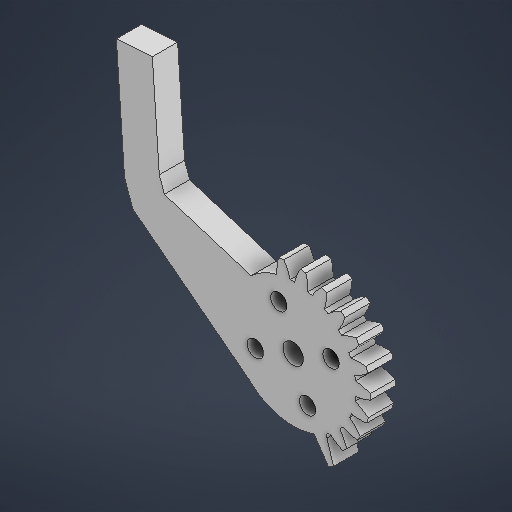
# Autodesk Inventor part: писюн 2
Saved by Autodesk Inventor 2025 (Build 290162000, 162)
## iProperties
Created: 2024-12-28
Part Number: писюн 2
Material: Типовые
Document SubType Name: Modeling
Designer: Phantom
Density: 1 g/cm^3
Appearance: По умолчанию
Author: Phantom
Autodesk Inventor part; units mm, degrees
(part 1 of 4)
ref_plane "YZ Plane" through (0, 0, 0) normal (1, 0, 0) x (0, 1, 0)
ref_plane "XZ Plane" through (0, 0, 0) normal (0, 1, 0) x (-1, 0, 0)
ref_plane "XY Plane" through (0, 0, 0) normal (0, 0, 1) x (1, 0, 0)
sketch "Эскиз1" plane through (0, 0, 0) normal (0, 0, 1) x (1, 0, 0)
  arc A0 (25.3405, 9.161) -> (8.4316, -5.5092) centre (48.8211, -34.9827) ccw
  arc A1 (16.1963, 14.3431) -> (25.3405, 9.161) centre (40.8164, 47.1281) ccw
  arc A2 (16.1963, 14.3431) -> (-11.1891, 14.3431) centre (2.5036, -3.8906) ccw
  line L0 (-11.1891, 14.3431) -> (-11.0924, 14.1698)
  line L1 (-11.0924, 14.1698) -> (-10.8798, 13.8428)
  line L2 (-10.8798, 13.8428) -> (-10.6476, 13.5415)
  line L3 (-10.6476, 13.5415) -> (-10.3902, 13.2744)
  line L4 (-10.3902, 13.2744) -> (-10.0964, 13.0589)
  line L5 (-10.0964, 13.0589) -> (-9.8198, 12.8188)
  line L6 (-9.8198, 12.8188) -> (-9.6918, 12.6838)
  line L7 (-9.6918, 12.6838) -> (-9.5723, 12.5363)
  line L8 (-9.5723, 12.5363) -> (-9.4633, 12.3731)
  line L9 (-9.4633, 12.3731) -> (-9.3681, 12.1883)
  line L10 (-9.3681, 12.1883) -> (-9.3278, 12.0845)
  line L11 (-9.3278, 12.0845) -> (-9.2943, 11.9695)
  line L12 (-9.2943, 11.9695) -> (-9.2712, 11.8376)
  line L13 (-9.2712, 11.8376) -> (-9.2668, 11.6743)
  line L14 (-9.2668, 11.6743) -> (-9.3696, 11.329)
  line L15 (-9.3696, 11.329) -> (-9.7265, 10.6764)
  line L16 (-9.7265, 10.6764) -> (-10.0432, 10.0032)
  line L17 (-10.0432, 10.0032) -> (-10.2615, 9.7167)
  line L18 (-10.2615, 9.7167) -> (-10.3959, 9.6239)
  line L19 (-10.3959, 9.6239) -> (-10.5161, 9.5649)
  line L20 (-10.5161, 9.5649) -> (-10.6287, 9.5241)
  line L21 (-10.6287, 9.5241) -> (-10.7364, 9.4955)
  line L22 (-10.7364, 9.4955) -> (-10.9417, 9.4634)
  line L23 (-10.9417, 9.4634) -> (-11.1379, 9.4552)
  line L24 (-11.1379, 9.4552) -> (-11.3274, 9.4648)
  line L25 (-11.3274, 9.4648) -> (-11.5119, 9.4885)
  line L26 (-11.5119, 9.4885) -> (-11.8689, 9.5704)
  line L27 (-11.8689, 9.5704) -> (-12.2162, 9.6807)
  line L28 (-12.2162, 9.6807) -> (-12.5837, 9.731)
  line L29 (-12.5837, 9.731) -> (-12.964, 9.741)
  line L30 (-12.964, 9.741) -> (-13.3534, 9.7199)
  line L31 (-13.3534, 9.7199) -> (-13.7498, 9.6714)
  line L32 (-13.7498, 9.6714) -> (-14.1519, 9.5976)
  line L33 (-14.1519, 9.5976) -> (-14.5586, 9.4998)
  line L34 (-14.5586, 9.4998) -> (-14.9687, 9.3787)
  line L35 (-14.9687, 9.3787) -> (-15.3815, 9.2349)
  line L36 (-15.3815, 9.2349) -> (-15.796, 9.069)
  line L37 (-15.796, 9.069) -> (-16.1075, 8.9301)
  line L38 (-16.1075, 8.9301) -> (-16.4414, 6.8067)
  line L39 (-16.4414, 6.8067) -> (-16.1875, 6.579)
  line L40 (-16.1875, 6.579) -> (-15.8439, 6.2938)
  line L41 (-15.8439, 6.2938) -> (-15.4952, 6.0303)
  line L42 (-15.4952, 6.0303) -> (-15.142, 5.7892)
  line L43 (-15.142, 5.7892) -> (-14.785, 5.5713)
  line L44 (-14.785, 5.5713) -> (-14.425, 5.3776)
  line L45 (-14.425, 5.3776) -> (-14.0625, 5.2099)
  line L46 (-14.0625, 5.2099) -> (-13.6984, 5.0703)
  line L47 (-13.6984, 5.0703) -> (-13.3334, 4.963)
  line L48 (-13.3334, 4.963) -> (-12.9682, 4.8982)
  line L49 (-12.9682, 4.8982) -> (-12.6038, 4.8965)
  line L50 (-12.6038, 4.8965) -> (-12.2389, 4.8649)
  line L51 (-12.2389, 4.8649) -> (-12.056, 4.8309)
  line L52 (-12.056, 4.8309) -> (-11.8727, 4.7818)
  line L53 (-11.8727, 4.7818) -> (-11.6885, 4.7139)
  line L54 (-11.6885, 4.7139) -> (-11.5029, 4.6203)
  line L55 (-11.5029, 4.6203) -> (-11.4093, 4.56)
  line L56 (-11.4093, 4.56) -> (-11.3146, 4.4866)
  line L57 (-11.3146, 4.4866) -> (-11.2183, 4.3936)
  line L58 (-11.2183, 4.3936) -> (-11.1188, 4.264)
  line L59 (-11.1188, 4.264) -> (-10.999, 3.9243)
  line L60 (-10.999, 3.9243) -> (-10.9042, 3.1865)
  line L61 (-10.9042, 3.1865) -> (-10.7647, 2.4558)
  line L62 (-10.7647, 2.4558) -> (-10.7729, 2.0956)
  line L63 (-10.7729, 2.0956) -> (-10.8272, 1.9416)
  line L64 (-10.8272, 1.9416) -> (-10.8897, 1.8232)
  line L65 (-10.8897, 1.8232) -> (-10.9568, 1.724)
  line L66 (-10.9568, 1.724) -> (-11.0271, 1.6375)
  line L67 (-11.0271, 1.6375) -> (-11.1743, 1.4909)
  line L68 (-11.1743, 1.4909) -> (-11.3282, 1.369)
  line L69 (-11.3282, 1.369) -> (-11.4872, 1.2653)
  line L70 (-11.4872, 1.2653) -> (-11.6504, 1.1761)
  line L71 (-11.6504, 1.1761) -> (-11.9874, 1.0325)
  line L72 (-11.9874, 1.0325) -> (-12.3332, 0.9175)
  line L73 (-12.3332, 0.9175) -> (-12.66, 0.7423)
  line L74 (-12.66, 0.7423) -> (-12.9736, 0.5268)
  line L75 (-12.9736, 0.5268) -> (-13.2762, 0.2808)
  line L76 (-13.2762, 0.2808) -> (-13.5684, 0.0086)
  line L77 (-13.5684, 0.0086) -> (-13.8504, -0.2874)
  line L78 (-13.8504, -0.2874) -> (-14.1218, -0.6056)
  line L79 (-14.1218, -0.6056) -> (-14.3824, -0.9447)
  line L80 (-14.3824, -0.9447) -> (-14.6319, -1.3036)
  line L81 (-14.6319, -1.3036) -> (-14.8697, -1.6815)
  line L82 (-14.8697, -1.6815) -> (-15.0401, -1.9769)
  line L83 (-15.0401, -1.9769) -> (-14.0621, -3.891)
  line L84 (-14.0621, -3.891) -> (-13.7228, -3.9261)
  line L85 (-13.7228, -3.9261) -> (-13.2773, -3.9548)
  line L86 (-13.2773, -3.9548) -> (-12.8403, -3.963)
  line L87 (-12.8403, -3.963) -> (-12.4128, -3.9505)
  line L88 (-12.4128, -3.9505) -> (-11.9959, -3.917)
  line L89 (-11.9959, -3.917) -> (-11.5908, -3.862)
  line L90 (-11.5908, -3.862) -> (-11.199, -3.7847)
  line L91 (-11.199, -3.7847) -> (-10.8224, -3.6836)
  line L92 (-10.8224, -3.6836) -> (-10.464, -3.5558)
  line L93 (-10.464, -3.5558) -> (-10.1304, -3.3936)
  line L94 (-10.1304, -3.3936) -> (-9.8347, -3.1808)
  line L95 (-9.8347, -3.1808) -> (-9.5209, -2.9918)
  line L96 (-9.5209, -2.9918) -> (-9.353, -2.9118)
  line L97 (-9.353, -2.9118) -> (-9.1758, -2.8438)
  line L98 (-9.1758, -2.8438) -> (-8.9868, -2.7905)
  line L99 (-8.9868, -2.7905) -> (-8.7817, -2.7571)
  line L100 (-8.7817, -2.7571) -> (-8.6705, -2.7509)
  line L101 (-8.6705, -2.7509) -> (-8.5508, -2.7546)
  line L102 (-8.5508, -2.7546) -> (-8.4182, -2.7733)
  line L103 (-8.4182, -2.7733) -> (-8.2615, -2.8196)
  line L104 (-8.2615, -2.8196) -> (-7.9649, -3.024)
  line L105 (-7.9649, -3.024) -> (-7.4545, -3.5652)
  line L106 (-7.4545, -3.5652) -> (-6.9122, -4.0744)
  line L107 (-6.9122, -4.0744) -> (-6.7071, -4.3705)
  line L108 (-6.7071, -4.3705) -> (-6.6604, -4.5271)
  line L109 (-6.6604, -4.5271) -> (-6.6415, -4.6596)
  line L110 (-6.6415, -4.6596) -> (-6.6374, -4.7793)
  line L111 (-6.6374, -4.7793) -> (-6.6435, -4.8906)
  line L112 (-6.6435, -4.8906) -> (-6.6764, -5.0958)
  line L113 (-6.6764, -5.0958) -> (-6.7292, -5.2848)
  line L114 (-6.7292, -5.2848) -> (-6.7969, -5.4622)
  line L115 (-6.7969, -5.4622) -> (-6.8765, -5.6303)
  line L116 (-6.8765, -5.6303) -> (-7.0647, -5.9445)
  line L117 (-7.0647, -5.9445) -> (-7.2769, -6.2407)
  line L118 (-7.2769, -6.2407) -> (-7.4384, -6.5746)
  line L119 (-7.4384, -6.5746) -> (-7.5654, -6.9333)
  line L120 (-7.5654, -6.9333) -> (-7.6656, -7.3102)
  line L121 (-7.6656, -7.3102) -> (-7.742, -7.7022)
  line L122 (-7.742, -7.7022) -> (-7.7961, -8.1074)
  line L123 (-7.7961, -8.1074) -> (-7.8287, -8.5243)
  line L124 (-7.8287, -8.5243) -> (-7.8403, -8.9518)
  line L125 (-7.8403, -8.9518) -> (-7.8311, -9.3888)
  line L126 (-7.8311, -9.3888) -> (-7.8013, -9.8343)
  line L127 (-7.8013, -9.8343) -> (-7.7656, -10.1735)
  line L128 (-7.7656, -10.1735) -> (-5.8492, -11.1472)
  line L129 (-5.8492, -11.1472) -> (-5.5542, -10.9761)
  line L130 (-5.5542, -10.9761) -> (-5.1768, -10.7375)
  line L131 (-5.1768, -10.7375) -> (-4.8185, -10.4872)
  line L132 (-4.8185, -10.4872) -> (-4.48, -10.2258)
  line L133 (-4.48, -10.2258) -> (-4.1624, -9.9537)
  line L134 (-4.1624, -9.9537) -> (-3.867, -9.6711)
  line L135 (-3.867, -9.6711) -> (-3.5955, -9.3782)
  line L136 (-3.5955, -9.3782) -> (-3.3502, -9.0751)
  line L137 (-3.3502, -9.0751) -> (-3.1354, -8.7611)
  line L138 (-3.1354, -8.7611) -> (-2.9609, -8.4338)
  line L139 (-2.9609, -8.4338) -> (-2.8467, -8.0877)
  line L140 (-2.8467, -8.0877) -> (-2.7039, -7.7505)
  line L141 (-2.7039, -7.7505) -> (-2.615, -7.5871)
  line L142 (-2.615, -7.5871) -> (-2.5117, -7.4278)
  line L143 (-2.5117, -7.4278) -> (-2.3901, -7.2737)
  line L144 (-2.3901, -7.2737) -> (-2.2438, -7.1261)
  line L145 (-2.2438, -7.1261) -> (-2.1575, -7.0556)
  line L146 (-2.1575, -7.0556) -> (-2.0585, -6.9883)
  line L147 (-2.0585, -6.9883) -> (-1.9402, -6.9255)
  line L148 (-1.9402, -6.9255) -> (-1.7863, -6.8709)
  line L149 (-1.7863, -6.8709) -> (-1.4262, -6.8619)
  line L150 (-1.4262, -6.8619) -> (-0.6951, -6.9997)
  line L151 (-0.6951, -6.9997) -> (0.0429, -7.0929)
  line L152 (0.0429, -7.0929) -> (0.3829, -7.2119)
  line L153 (0.3829, -7.2119) -> (0.5127, -7.3112)
  line L154 (0.5127, -7.3112) -> (0.6059, -7.4072)
  line L155 (0.6059, -7.4072) -> (0.6795, -7.5017)
  line L156 (0.6795, -7.5017) -> (0.74, -7.5953)
  line L157 (0.74, -7.5953) -> (0.834, -7.7806)
  line L158 (0.834, -7.7806) -> (0.9024, -7.9646)
  line L159 (0.9024, -7.9646) -> (0.9519, -8.1479)
  line L160 (0.9519, -8.1479) -> (0.9863, -8.3307)
  line L161 (0.9863, -8.3307) -> (1.0187, -8.6955)
  line L162 (1.0187, -8.6955) -> (1.0212, -9.0599)
  line L163 (1.0212, -9.0599) -> (1.0869, -9.4249)
  line L164 (1.0869, -9.4249) -> (1.1949, -9.7897)
  line L165 (1.1949, -9.7897) -> (1.3353, -10.1535)
  line L166 (1.3353, -10.1535) -> (1.5039, -10.5156)
  line L167 (1.5039, -10.5156) -> (1.6983, -10.8752)
  line L168 (1.6983, -10.8752) -> (1.9171, -11.2317)
  line L169 (1.9171, -11.2317) -> (2.159, -11.5843)
  line L170 (2.159, -11.5843) -> (2.4233, -11.9325)
  line L171 (2.4233, -11.9325) -> (2.7092, -12.2754)
  line L172 (2.7092, -12.2754) -> (2.9375, -12.5288)
  line L173 (2.9375, -12.5288) -> (5.0602, -12.1901)
  line L174 (5.0602, -12.1901) -> (5.1983, -11.8783)
  line L175 (5.1983, -11.8783) -> (5.3633, -11.4634)
  line L176 (5.3633, -11.4634) -> (5.5062, -11.0504)
  line L177 (5.5062, -11.0504) -> (5.6263, -10.6399)
  line L178 (5.6263, -10.6399) -> (5.7233, -10.2331)
  line L179 (5.7233, -10.2331) -> (5.7962, -9.8308)
  line L180 (5.7962, -9.8308) -> (5.8437, -9.4343)
  line L181 (5.8437, -9.4343) -> (5.864, -9.0449)
  line L182 (5.864, -9.0449) -> (5.8532, -8.6645)
  line L183 (5.8532, -8.6645) -> (5.802, -8.2972)
  line L184 (5.802, -8.2972) -> (5.691, -7.9502)
  line L185 (5.691, -7.9502) -> (5.6083, -7.5933)
  line L186 (5.6083, -7.5933) -> (5.5841, -7.4089)
  line L187 (5.5841, -7.4089) -> (5.5741, -7.2193)
  line L188 (5.5741, -7.2193) -> (5.5818, -7.0232)
  line L189 (5.5818, -7.0232) -> (5.6135, -6.8178)
  line L190 (5.6135, -6.8178) -> (5.6419, -6.7101)
  line L191 (5.6419, -6.7101) -> (5.6824, -6.5974)
  line L192 (5.6824, -6.5974) -> (5.7412, -6.4771)
  line L193 (5.7412, -6.4771) -> (5.8336, -6.3424)
  line L194 (5.8336, -6.3424) -> (6.1197, -6.1235)
  line L195 (6.1197, -6.1235) -> (6.7921, -5.8052)
  line L196 (6.7921, -5.8052) -> (7.444, -5.4468)
  line L197 (7.444, -5.4468) -> (7.789, -5.3433)
  line L198 (7.789, -5.3433) -> (7.9523, -5.3473)
  line L199 (7.9523, -5.3473) -> (8.0842, -5.3702)
  line L200 (8.0842, -5.3702) -> (8.1993, -5.4034)
  line L201 (8.1993, -5.4034) -> (8.3032, -5.4435)
  line L202 (8.3032, -5.4435) -> (8.4316, -5.5092)
  circle A3 centre (-5.9559, 8.675) radius 1.6
  circle A4 centre (-2.3455, -2.0471) radius 1.6
  circle A5 centre (8.3767, 1.5633) radius 1.6
  circle A6 centre (4.7663, 12.2855) radius 1.6
  circle A7 centre (1.2104, 5.1192) radius 2.5
  line L203 (-13.3615, -49.398) -> (-13.2922, -49.3107)
  line L204 (-13.2922, -49.3107) -> (-13.2099, -49.2238)
  line L205 (-13.2099, -49.2238) -> (-13.1078, -49.1372)
  line L206 (-9.6165, -50.932) -> (-9.433, -51.2653)
  line L207 (-9.433, -51.2653) -> (-9.3025, -51.4628)
  line L208 (-9.7587, -50.5894) -> (-9.6165, -50.932)
  line L209 (-10.4254, -49.1402) -> (-10.3463, -49.2187)
  line L210 (-10.3463, -49.2187) -> (-10.2149, -49.3797)
  line L211 (-10.2149, -49.3797) -> (-10.1088, -49.5448)
  line L212 (-10.1088, -49.5448) -> (-10.0213, -49.7133)
  line L213 (-10.0213, -49.7133) -> (-9.9486, -49.8845)
  line L214 (-9.9486, -49.8845) -> (-9.8389, -50.234)
  line L215 (-9.8389, -50.234) -> (-9.7587, -50.5894)
  circle A8 centre (-5.8233, -40.9429) radius 1.6
  arc A9 (11.8073, -35.0555) -> (-9.3025, -51.4628) centre (30.819, -81.3) ccw
  line L216 (-13.8831, -51.1857) -> (-13.7825, -50.8287)
  line L217 (-13.7825, -50.8287) -> (-13.7449, -50.4663)
  line L218 (-13.7449, -50.4663) -> (-13.6775, -50.1063)
  line L219 (-13.6775, -50.1063) -> (-13.6256, -49.9276)
  line L220 (-13.6256, -49.9276) -> (-13.5587, -49.75)
  line L221 (-13.5587, -49.75) -> (-13.4729, -49.5734)
  line L222 (-13.4729, -49.5734) -> (-13.3615, -49.398)
  line L223 (-11.1347, -48.8769) -> (-10.7771, -48.9205)
  line L224 (-11.8756, -48.9436) -> (-11.1347, -48.8769)
  line L225 (-12.6192, -48.9652) -> (-11.8756, -48.9436)
  line L226 (-10.7771, -48.9205) -> (-10.6291, -48.9898)
  line L227 (-10.6291, -48.9898) -> (-10.5175, -49.0637)
  line L228 (-10.5175, -49.0637) -> (-10.4254, -49.1402)
  line L229 (-13.1078, -49.1372) -> (-12.9691, -49.0509)
  line L230 (-12.9691, -49.0509) -> (-12.6192, -48.9652)
  line L231 (-15.7727, -53.8665) -> (-15.455, -53.5527)
  line L232 (-15.455, -53.5527) -> (-15.1584, -53.2317)
  line L233 (-15.1584, -53.2317) -> (-14.8836, -52.904)
  line L234 (-14.8836, -52.904) -> (-14.6315, -52.5703)
  line L235 (-14.0258, -51.5384) -> (-13.8831, -51.1857)
  line L236 (-14.2006, -51.887) -> (-14.0258, -51.5384)
  line L237 (-14.4034, -52.2311) -> (-14.2006, -51.887)
  line L238 (-14.6315, -52.5703) -> (-14.4034, -52.2311)
  line L239 (-16.0243, -54.0967) -> (-15.7727, -53.8665)
  line L240 (-18.165, -48.7455) -> (-18.2068, -48.9267)
  line L241 (-18.2068, -48.9267) -> (-18.3236, -49.2739)
  line L242 (-18.3236, -49.2739) -> (-18.4675, -49.6086)
  line L243 (-18.4675, -49.6086) -> (-18.5539, -49.9694)
  line L244 (-18.5539, -49.9694) -> (-18.6013, -50.3469)
  line L245 (-18.1045, -53.555) -> (-16.0243, -54.0967)
  line L246 (-18.2119, -53.2313) -> (-18.1045, -53.555)
  line L247 (-18.3362, -52.8024) -> (-18.2119, -53.2313)
  line L248 (-18.4385, -52.3775) -> (-18.3362, -52.8024)
  line L249 (-18.5186, -51.9574) -> (-18.4385, -52.3775)
  line L250 (-18.5758, -51.5431) -> (-18.5186, -51.9574)
  line L251 (-18.6096, -51.1357) -> (-18.5758, -51.5431)
  line L252 (-18.6013, -50.3469) -> (-18.6187, -50.7364)
  line L253 (-18.6187, -50.7364) -> (-18.6096, -51.1357)
  line L254 (-19.827, -46.6133) -> (-19.2128, -47.0328)
  line L255 (-19.2128, -47.0328) -> (-18.5742, -47.4144)
  line L256 (-18.5742, -47.4144) -> (-18.3105, -47.6599)
  line L257 (-18.3105, -47.6599) -> (-18.2315, -47.8028)
  line L258 (-18.2315, -47.8028) -> (-18.1846, -47.9283)
  line L259 (-18.1846, -47.9283) -> (-18.1551, -48.0444)
  line L260 (-18.1551, -48.0444) -> (-18.1373, -48.1543)
  line L261 (-18.1373, -48.1543) -> (-18.1256, -48.3618)
  line L262 (-18.1256, -48.3618) -> (-18.1368, -48.5578)
  line L263 (-18.1368, -48.5578) -> (-18.165, -48.7455)
  line L264 (-24.325, -43.2978) -> (-24.6235, -43.5101)
  line L265 (-24.1846, -43.1758) -> (-24.325, -43.2978)
  line L266 (-24.0514, -43.0405) -> (-24.1846, -43.1758)
  line L267 (-23.9271, -42.8885) -> (-24.0514, -43.0405)
  line L268 (-23.8146, -42.7138) -> (-23.9271, -42.8885)
  line L269 (-23.7645, -42.6143) -> (-23.8146, -42.7138)
  line L270 (-23.7201, -42.5031) -> (-23.7645, -42.6143)
  line L271 (-23.6843, -42.3741) -> (-23.7201, -42.5031)
  line L272 (-23.6642, -42.2119) -> (-23.6843, -42.3741)
  line L273 (-26.3323, -35.144) -> (-26.6951, -35.1105)
  line L274 (-25.966, -35.1478) -> (-26.3323, -35.144)
  line L275 (-25.7807, -35.1315) -> (-25.966, -35.1478)
  line L276 (-25.5935, -35.1004) -> (-25.7807, -35.1315)
  line L277 (-25.4036, -35.0505) -> (-25.5935, -35.1004)
  line L278 (-25.2099, -34.9752) -> (-25.4036, -35.0505)
  line L279 (-25.1108, -34.9243) -> (-25.2099, -34.9752)
  line L280 (-25.0095, -34.8603) -> (-25.1108, -34.9243)
  line L281 (-22.4775, -47.8682) -> (-22.1548, -47.6668)
  line L282 (-22.1548, -47.6668) -> (-21.8636, -47.4371)
  line L283 (-25.6882, -39.8199) -> (-25.5023, -39.814)
  line L284 (-26.0514, -39.867) -> (-25.6882, -39.8199)
  line L285 (-26.7783, -39.958) -> (-26.4077, -39.9433)
  line L286 (-26.4077, -39.9433) -> (-26.0514, -39.867)
  line L287 (-25.5023, -39.814) -> (-25.3126, -39.8228)
  line L288 (-25.3126, -39.8228) -> (-25.1182, -39.8498)
  line L289 (-25.1182, -39.8498) -> (-24.9169, -39.9016)
  line L290 (-24.9169, -39.9016) -> (-24.8125, -39.9405)
  line L291 (-24.8125, -39.9405) -> (-24.7044, -39.9919)
  line L292 (-24.7044, -39.9919) -> (-24.5904, -40.0623)
  line L293 (-24.5904, -40.0623) -> (-24.4655, -40.1675)
  line L294 (-24.4655, -40.1675) -> (-24.2759, -40.4738)
  line L295 (-24.2759, -40.4738) -> (-24.0256, -41.1743)
  line L296 (-24.0256, -41.1743) -> (-23.7332, -41.8584)
  line L297 (-23.7332, -41.8584) -> (-23.6642, -42.2119)
  line L298 (-24.2664, -32.892) -> (-24.4757, -33.6058)
  line L299 (-24.2398, -32.5327) -> (-24.2664, -32.892)
  line L300 (-24.279, -32.3741) -> (-24.2398, -32.5327)
  line L301 (-24.3298, -32.2502) -> (-24.279, -32.3741)
  line L302 (-24.3871, -32.145) -> (-24.3298, -32.2502)
  line L303 (-24.4487, -32.0522) -> (-24.3871, -32.145)
  line L304 (-24.5811, -31.892) -> (-24.4487, -32.0522)
  line L305 (-24.8708, -31.6373) -> (-24.7225, -31.7559)
  line L306 (-24.7225, -31.7559) -> (-24.5811, -31.892)
  circle A10 centre (-19.3845, -32.452) radius 1.6
  arc A11 (3.2188, -28.9967) -> (-27.6302, -28.9967) centre (-12.2057, -45.7908) ccw
  circle A12 centre (-8.3584, -29.9169) radius 1.6
  line L307 (-24.9367, -43.6962) -> (-25.2186, -43.9373)
  line L308 (-25.2186, -43.9373) -> (-25.4788, -44.2149)
  line L309 (-25.4788, -44.2149) -> (-25.7219, -44.5198)
  line L310 (-25.7219, -44.5198) -> (-25.9492, -44.8482)
  line L311 (-25.9492, -44.8482) -> (-26.1614, -45.1976)
  line L312 (-26.1614, -45.1976) -> (-26.3585, -45.5664)
  line L313 (-26.3585, -45.5664) -> (-26.5407, -45.9534)
  line L314 (-24.6235, -43.5101) -> (-24.9367, -43.6962)
  line L315 (-27.0648, -35.1399) -> (-27.4385, -35.2114)
  line L316 (-24.9047, -34.777) -> (-25.0095, -34.8603)
  line L317 (-24.7932, -34.6577) -> (-24.9047, -34.777)
  line L318 (-24.6412, -34.3311) -> (-24.7932, -34.6577)
  line L319 (-28.3264, -39.674) -> (-27.9333, -39.7862)
  circle A13 centre (-12.6039, -36.6975) radius 2.5
  line L320 (-26.6951, -35.1105) -> (-27.0648, -35.1399)
  line L321 (-22.8239, -48.0475) -> (-22.4775, -47.8682)
  line L322 (-23.1901, -48.2067) -> (-22.8239, -48.0475)
  line L323 (-23.5741, -48.347) -> (-23.1901, -48.2067)
  line L324 (-23.9742, -48.4688) -> (-23.5741, -48.347)
  line L325 (-24.3891, -48.5724) -> (-23.9742, -48.4688)
  line L326 (-24.8178, -48.6578) -> (-24.3891, -48.5724)
  line L327 (-25.2592, -48.7249) -> (-24.8178, -48.6578)
  line L328 (-26.7077, -46.3573) -> (-26.8592, -46.7773)
  line L329 (-26.8592, -46.7773) -> (-26.9625, -47.1023)
  line L330 (-26.9625, -47.1023) -> (-25.5981, -48.7632)
  line L331 (-25.5981, -48.7632) -> (-25.2592, -48.7249)
  line L332 (-24.4757, -33.6058) -> (-24.6412, -34.3311)
  line L333 (-27.4385, -35.2114) -> (-27.8144, -35.3153)
  line L334 (-27.8144, -35.3153) -> (-28.1913, -35.4473)
  line L335 (-28.5684, -35.6053) -> (-28.9447, -35.7878)
  line L336 (-28.9447, -35.7878) -> (-29.3195, -35.9938)
  line L337 (-29.3195, -35.9938) -> (-29.692, -36.2224)
  line L338 (-29.692, -36.2224) -> (-30.0614, -36.4731)
  line L339 (-30.0614, -36.4731) -> (-30.3361, -36.6753)
  line L340 (-28.1913, -35.4473) -> (-28.5684, -35.6053)
  line L341 (-25.0246, -31.5328) -> (-24.8708, -31.6373)
  line L342 (-25.3462, -31.3574) -> (-25.0246, -31.5328)
  line L343 (-25.9877, -31.0037) -> (-25.6793, -31.2097)
  line L344 (-26.279, -30.759) -> (-25.9877, -31.0037)
  line L345 (-26.5565, -30.485) -> (-26.279, -30.759)
  line L346 (-26.8212, -30.1859) -> (-26.5565, -30.485)
  line L347 (-27.0732, -29.864) -> (-26.8212, -30.1859)
  line L348 (-27.3127, -29.5212) -> (-27.0732, -29.864)
  line L349 (-27.5395, -29.1586) -> (-27.3127, -29.5212)
  line L350 (-27.6302, -28.9967) -> (-27.5395, -29.1586)
  line L351 (-25.6793, -31.2097) -> (-25.3462, -31.3574)
  line L352 (-30.3361, -36.6753) -> (-30.2085, -38.8211)
  line L353 (-30.2085, -38.8211) -> (-29.9118, -38.9893)
  line L354 (-29.9118, -38.9893) -> (-29.5152, -39.1944)
  line L355 (-29.5152, -39.1944) -> (-29.1183, -39.3773)
  line L356 (-29.1183, -39.3773) -> (-28.7217, -39.5374)
  line L357 (-28.7217, -39.5374) -> (-28.3264, -39.674)
  line L358 (-27.9333, -39.7862) -> (-27.5434, -39.8726)
  line L359 (-27.5434, -39.8726) -> (-27.1579, -39.9312)
  line L360 (-26.5407, -45.9534) -> (-26.7077, -46.3573)
  line L361 (-27.1579, -39.9312) -> (-26.7783, -39.958)
  line L362 (-21.8636, -47.4371) -> (-21.6201, -47.166)
  line L363 (-21.6201, -47.166) -> (-21.354, -46.9143)
  line L364 (-21.354, -46.9143) -> (-21.207, -46.8003)
  line L365 (-21.207, -46.8003) -> (-21.0484, -46.696)
  line L366 (-21.0484, -46.696) -> (-20.8752, -46.6035)
  line L367 (-20.682, -46.5271) -> (-20.5747, -46.4972)
  circle A14 centre (-16.8493, -43.478) radius 1.6
  line L368 (-20.1605, -46.4769) -> (-19.827, -46.6133)
  line L369 (-20.3234, -46.4652) -> (-20.1605, -46.4769)
  line L370 (-20.4569, -46.4753) -> (-20.3234, -46.4652)
  line L371 (-20.5747, -46.4972) -> (-20.4569, -46.4753)
  line L372 (-20.8752, -46.6035) -> (-20.682, -46.5271)
  arc A15 (3.2188, -28.9967) -> (11.8073, -35.0555) centre (30.9527, 1.1999) ccw
  point P0 (0, 0)
  point P1 (-20.9679, -17.3277)
  point P2 (-6.0215, -34.9827)
  constraints: 746 end point, 16 centre point, 12 point on circle
extrude "Выдавливание1" add sketch "Эскиз1" along normal blind 5 contours L222 L221 L220 L219 L218 L217 L216 L235 L236 L237 L238 L234 L233 L232 L231 L239 L245 L246 L247 L248 L249 L250 L251 L253 L252 L244 L243 L242 L241 L240 L263 L262 L261 L260 L259 L258 L257 L256 L255 L254 L368 L369 L370 L371 L367 L372 L366 L365 L364 L363 L362 L282 L281 L321 L322 L323 L324 L325 L326 L327 L331 L330 L329 L328 L360 L313 L312 L311 L310 L309 L308 L307 L314 L264 L265 L266 L267 L268 L269 L270 L271 L272 L297 L296 L295 L294 L293 L292 L291 L290 L289 L288 L287 L283 L284 L286 L285 L361 L359 L358 L319 L357 L356 L355 L354 L353 L352 L339 L338 L337 L336 L335 L340 L334 L333 L315 L320 L273 L274 L275 L276 L277 L278 L279 L280 L316 L317 L318 L332 L298 L299 L300 L301 L302 L303 L304 L306 L305 L341 L342 L351 L343 L344 L345 L346 L347 L348 L349 L350 A11 A15 A9 L207 L206 L208 L215 L214 L213 L212 L211 L210 L209 L228 L227 L226 L223 L224 L225 L230 L229 L205 L204 L203
sketch "Эскиз2" plane through (0, 0, 0) normal (0, 0, -1) x (-1, 0, 0)
  line L0 (-8.3032, -5.4435) -> (-8.4316, -5.5092) projected
  line L1 (-8.4316, -5.5092) -> (-25.3405, -5.5092)
  line L2 (11.1891, 14.3431) -> (11.0924, 14.1698) projected
  arc A0 (11.1891, 14.3431) -> (-16.1963, 14.3431) centre (-2.5036, -3.8906) ccw projected
  arc A1 (-25.3405, 9.161) -> (-16.1963, 14.3431) centre (-40.8164, 47.1281) ccw projected
  arc A2 (-8.4316, -5.5092) -> (-25.3405, 9.161) centre (-48.8211, -34.9827) ccw projected
  line L3 (-8.3032, -5.4435) -> (-8.4316, -5.5092) projected
  line L4 (-8.1993, -5.4034) -> (-8.3032, -5.4435) projected
  line L5 (-8.0842, -5.3702) -> (-8.1993, -5.4034) projected
  line L6 (-7.9523, -5.3473) -> (-8.0842, -5.3702) projected
  line L7 (-7.789, -5.3433) -> (-7.9523, -5.3473) projected
  line L8 (-7.444, -5.4468) -> (-7.789, -5.3433) projected
  line L9 (-6.7921, -5.8052) -> (-7.444, -5.4468) projected
  line L10 (-6.1197, -6.1235) -> (-6.7921, -5.8052) projected
  line L11 (-5.8336, -6.3424) -> (-6.1197, -6.1235) projected
  line L12 (-5.7412, -6.4771) -> (-5.8336, -6.3424) projected
  line L13 (-5.6824, -6.5974) -> (-5.7412, -6.4771) projected
  line L14 (-5.6419, -6.7101) -> (-5.6824, -6.5974) projected
  line L15 (-5.6135, -6.8178) -> (-5.6419, -6.7101) projected
  line L16 (-5.5818, -7.0232) -> (-5.6135, -6.8178) projected
  line L17 (-5.5741, -7.2193) -> (-5.5818, -7.0232) projected
  line L18 (-5.5841, -7.4089) -> (-5.5741, -7.2193) projected
  line L19 (-5.6083, -7.5933) -> (-5.5841, -7.4089) projected
  line L20 (-5.691, -7.9502) -> (-5.6083, -7.5933) projected
  line L21 (-5.802, -8.2972) -> (-5.691, -7.9502) projected
  line L22 (-5.8532, -8.6645) -> (-5.802, -8.2972) projected
  line L23 (-5.864, -9.0449) -> (-5.8532, -8.6645) projected
  line L24 (-5.8437, -9.4343) -> (-5.864, -9.0449) projected
  line L25 (-5.7962, -9.8308) -> (-5.8437, -9.4343) projected
  line L26 (-5.7233, -10.2331) -> (-5.7962, -9.8308) projected
  line L27 (-5.6263, -10.6399) -> (-5.7233, -10.2331) projected
  line L28 (-5.5062, -11.0504) -> (-5.6263, -10.6399) projected
  line L29 (-5.3633, -11.4634) -> (-5.5062, -11.0504) projected
  line L30 (-5.1983, -11.8783) -> (-5.3633, -11.4634) projected
  line L31 (-5.0602, -12.1901) -> (-5.1983, -11.8783) projected
  line L32 (-2.9375, -12.5288) -> (-5.0602, -12.1901) projected
  line L33 (-2.7092, -12.2754) -> (-2.9375, -12.5288) projected
  line L34 (-2.4233, -11.9325) -> (-2.7092, -12.2754) projected
  line L35 (-2.159, -11.5843) -> (-2.4233, -11.9325) projected
  line L36 (-1.9171, -11.2317) -> (-2.159, -11.5843) projected
  line L37 (-1.6983, -10.8752) -> (-1.9171, -11.2317) projected
  line L38 (-1.5039, -10.5156) -> (-1.6983, -10.8752) projected
  line L39 (-1.3353, -10.1535) -> (-1.5039, -10.5156) projected
  line L40 (-1.1949, -9.7897) -> (-1.3353, -10.1535) projected
  line L41 (-1.0869, -9.4249) -> (-1.1949, -9.7897) projected
  line L42 (-1.0212, -9.0599) -> (-1.0869, -9.4249) projected
  line L43 (-1.0187, -8.6955) -> (-1.0212, -9.0599) projected
  line L44 (-0.9863, -8.3307) -> (-1.0187, -8.6955) projected
  line L45 (-0.9519, -8.1479) -> (-0.9863, -8.3307) projected
  line L46 (-0.9024, -7.9646) -> (-0.9519, -8.1479) projected
  line L47 (-0.834, -7.7806) -> (-0.9024, -7.9646) projected
  line L48 (-0.74, -7.5953) -> (-0.834, -7.7806) projected
  line L49 (-0.6795, -7.5017) -> (-0.74, -7.5953) projected
  line L50 (-0.6059, -7.4072) -> (-0.6795, -7.5017) projected
  line L51 (-0.5127, -7.3112) -> (-0.6059, -7.4072) projected
  line L52 (-0.3829, -7.2119) -> (-0.5127, -7.3112) projected
  line L53 (-0.0429, -7.0929) -> (-0.3829, -7.2119) projected
  line L54 (0.6951, -6.9997) -> (-0.0429, -7.0929) projected
  line L55 (1.4262, -6.8619) -> (0.6951, -6.9997) projected
  line L56 (1.7863, -6.8709) -> (1.4262, -6.8619) projected
  line L57 (1.9402, -6.9255) -> (1.7863, -6.8709) projected
  line L58 (2.0585, -6.9883) -> (1.9402, -6.9255) projected
  line L59 (2.1575, -7.0556) -> (2.0585, -6.9883) projected
  line L60 (2.2438, -7.1261) -> (2.1575, -7.0556) projected
  line L61 (2.3901, -7.2737) -> (2.2438, -7.1261) projected
  line L62 (2.5117, -7.4278) -> (2.3901, -7.2737) projected
  line L63 (2.615, -7.5871) -> (2.5117, -7.4278) projected
  line L64 (2.7039, -7.7505) -> (2.615, -7.5871) projected
  line L65 (2.8467, -8.0877) -> (2.7039, -7.7505) projected
  line L66 (2.9609, -8.4338) -> (2.8467, -8.0877) projected
  line L67 (3.1354, -8.7611) -> (2.9609, -8.4338) projected
  line L68 (3.3502, -9.0751) -> (3.1354, -8.7611) projected
  line L69 (3.5955, -9.3782) -> (3.3502, -9.0751) projected
  line L70 (3.867, -9.6711) -> (3.5955, -9.3782) projected
  line L71 (4.1624, -9.9537) -> (3.867, -9.6711) projected
  line L72 (4.48, -10.2258) -> (4.1624, -9.9537) projected
  line L73 (4.8185, -10.4872) -> (4.48, -10.2258) projected
  line L74 (5.1768, -10.7375) -> (4.8185, -10.4872) projected
  line L75 (5.5542, -10.9761) -> (5.1768, -10.7375) projected
  line L76 (5.8492, -11.1472) -> (5.5542, -10.9761) projected
  line L77 (7.7656, -10.1735) -> (5.8492, -11.1472) projected
  line L78 (7.8013, -9.8343) -> (7.7656, -10.1735) projected
  line L79 (7.8311, -9.3888) -> (7.8013, -9.8343) projected
  line L80 (7.8403, -8.9518) -> (7.8311, -9.3888) projected
  line L81 (7.8287, -8.5243) -> (7.8403, -8.9518) projected
  line L82 (7.7961, -8.1074) -> (7.8287, -8.5243) projected
  line L83 (7.742, -7.7022) -> (7.7961, -8.1074) projected
  line L84 (7.6656, -7.3102) -> (7.742, -7.7022) projected
  line L85 (7.5654, -6.9333) -> (7.6656, -7.3102) projected
  line L86 (7.4384, -6.5746) -> (7.5654, -6.9333) projected
  line L87 (7.2769, -6.2407) -> (7.4384, -6.5746) projected
  line L88 (7.0647, -5.9445) -> (7.2769, -6.2407) projected
  line L89 (6.8765, -5.6303) -> (7.0647, -5.9445) projected
  line L90 (6.7969, -5.4622) -> (6.8765, -5.6303) projected
  line L91 (6.7292, -5.2848) -> (6.7969, -5.4622) projected
  line L92 (6.6764, -5.0958) -> (6.7292, -5.2848) projected
  line L93 (6.6435, -4.8906) -> (6.6764, -5.0958) projected
  line L94 (6.6374, -4.7793) -> (6.6435, -4.8906) projected
  line L95 (6.6415, -4.6596) -> (6.6374, -4.7793) projected
  line L96 (6.6604, -4.5271) -> (6.6415, -4.6596) projected
  line L97 (6.7071, -4.3705) -> (6.6604, -4.5271) projected
  line L98 (6.9122, -4.0744) -> (6.7071, -4.3705) projected
  line L99 (7.4545, -3.5652) -> (6.9122, -4.0744) projected
  line L100 (7.9649, -3.024) -> (7.4545, -3.5652) projected
  line L101 (8.2615, -2.8196) -> (7.9649, -3.024) projected
  line L102 (8.4182, -2.7733) -> (8.2615, -2.8196) projected
  line L103 (8.5508, -2.7546) -> (8.4182, -2.7733) projected
  line L104 (8.6705, -2.7509) -> (8.5508, -2.7546) projected
  line L105 (8.7817, -2.7571) -> (8.6705, -2.7509) projected
  line L106 (8.9868, -2.7905) -> (8.7817, -2.7571) projected
  line L107 (9.1758, -2.8438) -> (8.9868, -2.7905) projected
  line L108 (9.353, -2.9118) -> (9.1758, -2.8438) projected
  line L109 (9.5209, -2.9918) -> (9.353, -2.9118) projected
  line L110 (9.8347, -3.1808) -> (9.5209, -2.9918) projected
  line L111 (10.1304, -3.3936) -> (9.8347, -3.1808) projected
  line L112 (10.464, -3.5558) -> (10.1304, -3.3936) projected
  line L113 (10.8224, -3.6836) -> (10.464, -3.5558) projected
  line L114 (11.199, -3.7847) -> (10.8224, -3.6836) projected
  line L115 (11.5908, -3.862) -> (11.199, -3.7847) projected
  line L116 (11.9959, -3.917) -> (11.5908, -3.862) projected
  line L117 (12.4128, -3.9505) -> (11.9959, -3.917) projected
  line L118 (12.8403, -3.963) -> (12.4128, -3.9505) projected
  line L119 (13.2773, -3.9548) -> (12.8403, -3.963) projected
  line L120 (13.7228, -3.9261) -> (13.2773, -3.9548) projected
  line L121 (14.0621, -3.891) -> (13.7228, -3.9261) projected
  line L122 (15.0401, -1.9769) -> (14.0621, -3.891) projected
  line L123 (14.8697, -1.6815) -> (15.0401, -1.9769) projected
  line L124 (14.6319, -1.3036) -> (14.8697, -1.6815) projected
  line L125 (14.3824, -0.9447) -> (14.6319, -1.3036) projected
  line L126 (14.1218, -0.6056) -> (14.3824, -0.9447) projected
  line L127 (13.8504, -0.2874) -> (14.1218, -0.6056) projected
  line L128 (13.5684, 0.0086) -> (13.8504, -0.2874) projected
  line L129 (13.2762, 0.2808) -> (13.5684, 0.0086) projected
  line L130 (12.9736, 0.5268) -> (13.2762, 0.2808) projected
  line L131 (12.66, 0.7423) -> (12.9736, 0.5268) projected
  line L132 (12.3332, 0.9175) -> (12.66, 0.7423) projected
  line L133 (11.9874, 1.0325) -> (12.3332, 0.9175) projected
  line L134 (11.6504, 1.1761) -> (11.9874, 1.0325) projected
  line L135 (11.4872, 1.2653) -> (11.6504, 1.1761) projected
  line L136 (11.3282, 1.369) -> (11.4872, 1.2653) projected
  line L137 (11.1743, 1.4909) -> (11.3282, 1.369) projected
  line L138 (11.0271, 1.6375) -> (11.1743, 1.4909) projected
  line L139 (10.9568, 1.724) -> (11.0271, 1.6375) projected
  line L140 (10.8897, 1.8232) -> (10.9568, 1.724) projected
  line L141 (10.8272, 1.9416) -> (10.8897, 1.8232) projected
  line L142 (10.7729, 2.0956) -> (10.8272, 1.9416) projected
  line L143 (10.7647, 2.4558) -> (10.7729, 2.0956) projected
  line L144 (10.9042, 3.1865) -> (10.7647, 2.4558) projected
  line L145 (10.999, 3.9243) -> (10.9042, 3.1865) projected
  line L146 (11.1188, 4.264) -> (10.999, 3.9243) projected
  line L147 (11.2183, 4.3936) -> (11.1188, 4.264) projected
  line L148 (11.3146, 4.4866) -> (11.2183, 4.3936) projected
  line L149 (11.4093, 4.56) -> (11.3146, 4.4866) projected
  line L150 (11.5029, 4.6203) -> (11.4093, 4.56) projected
  line L151 (11.6885, 4.7139) -> (11.5029, 4.6203) projected
  line L152 (11.8727, 4.7818) -> (11.6885, 4.7139) projected
  line L153 (12.056, 4.8309) -> (11.8727, 4.7818) projected
  line L154 (12.2389, 4.8649) -> (12.056, 4.8309) projected
  line L155 (12.6038, 4.8965) -> (12.2389, 4.8649) projected
  line L156 (12.9682, 4.8982) -> (12.6038, 4.8965) projected
  line L157 (13.3334, 4.963) -> (12.9682, 4.8982) projected
  line L158 (13.6984, 5.0703) -> (13.3334, 4.963) projected
  line L159 (14.0625, 5.2099) -> (13.6984, 5.0703) projected
  line L160 (14.425, 5.3776) -> (14.0625, 5.2099) projected
  line L161 (14.785, 5.5713) -> (14.425, 5.3776) projected
  line L162 (15.142, 5.7892) -> (14.785, 5.5713) projected
  line L163 (15.4952, 6.0303) -> (15.142, 5.7892) projected
  line L164 (15.8439, 6.2938) -> (15.4952, 6.0303) projected
  line L165 (16.1875, 6.579) -> (15.8439, 6.2938) projected
  line L166 (16.4414, 6.8067) -> (16.1875, 6.579) projected
  line L167 (16.1075, 8.9301) -> (16.4414, 6.8067) projected
  line L168 (15.796, 9.069) -> (16.1075, 8.9301) projected
  line L169 (15.3815, 9.2349) -> (15.796, 9.069) projected
  line L170 (14.9687, 9.3787) -> (15.3815, 9.2349) projected
  line L171 (14.5586, 9.4998) -> (14.9687, 9.3787) projected
  line L172 (14.1519, 9.5976) -> (14.5586, 9.4998) projected
  line L173 (13.7498, 9.6714) -> (14.1519, 9.5976) projected
  line L174 (13.3534, 9.7199) -> (13.7498, 9.6714) projected
  line L175 (12.964, 9.741) -> (13.3534, 9.7199) projected
  line L176 (12.5837, 9.731) -> (12.964, 9.741) projected
  line L177 (12.2162, 9.6807) -> (12.5837, 9.731) projected
  line L178 (11.8689, 9.5704) -> (12.2162, 9.6807) projected
  line L179 (11.5119, 9.4885) -> (11.8689, 9.5704) projected
  line L180 (11.3274, 9.4648) -> (11.5119, 9.4885) projected
  line L181 (11.1379, 9.4552) -> (11.3274, 9.4648) projected
  line L182 (10.9417, 9.4634) -> (11.1379, 9.4552) projected
  line L183 (10.7364, 9.4955) -> (10.9417, 9.4634) projected
  line L184 (10.6287, 9.5241) -> (10.7364, 9.4955) projected
  line L185 (10.5161, 9.5649) -> (10.6287, 9.5241) projected
  line L186 (10.3959, 9.6239) -> (10.5161, 9.5649) projected
  line L187 (10.2615, 9.7167) -> (10.3959, 9.6239) projected
  line L188 (10.0432, 10.0032) -> (10.2615, 9.7167) projected
  line L189 (9.7265, 10.6764) -> (10.0432, 10.0032) projected
  line L190 (9.3696, 11.329) -> (9.7265, 10.6764) projected
  line L191 (9.2668, 11.6743) -> (9.3696, 11.329) projected
  line L192 (9.2712, 11.8376) -> (9.2668, 11.6743) projected
  line L193 (9.2943, 11.9695) -> (9.2712, 11.8376) projected
  line L194 (9.3278, 12.0845) -> (9.2943, 11.9695) projected
  line L195 (9.3681, 12.1883) -> (9.3278, 12.0845) projected
  line L196 (9.4633, 12.3731) -> (9.3681, 12.1883) projected
  line L197 (9.5723, 12.5363) -> (9.4633, 12.3731) projected
  line L198 (9.6918, 12.6838) -> (9.5723, 12.5363) projected
  line L199 (9.8198, 12.8188) -> (9.6918, 12.6838) projected
  line L200 (10.0964, 13.0589) -> (9.8198, 12.8188) projected
  line L201 (10.3902, 13.2744) -> (10.0964, 13.0589) projected
  line L202 (10.6476, 13.5415) -> (10.3902, 13.2744) projected
  line L203 (10.8798, 13.8428) -> (10.6476, 13.5415) projected
  line L204 (11.0924, 14.1698) -> (10.8798, 13.8428) projected
  circle A3 centre (-8.3767, 1.5633) radius 1.6 projected
  circle A4 centre (2.3455, -2.0471) radius 1.6 projected
  circle A5 centre (5.9559, 8.675) radius 1.6 projected
  circle A6 centre (-4.7663, 12.2855) radius 1.6 projected
  circle A7 centre (-1.2104, 5.1192) radius 2.5 projected
  line L205 (-25.3405, 9.161) -> (-25.3405, -5.5092)
  line L206 (27.6302, -28.9967) -> (27.5395, -29.1586) projected
  line L207 (27.5395, -29.1586) -> (27.3127, -29.5212) projected
  line L208 (27.3127, -29.5212) -> (27.0732, -29.864) projected
  line L209 (27.0732, -29.864) -> (26.8212, -30.1859) projected
  line L210 (26.8212, -30.1859) -> (26.5565, -30.485) projected
  line L211 (26.5565, -30.485) -> (26.279, -30.759) projected
  line L212 (26.279, -30.759) -> (25.9877, -31.0037) projected
  line L213 (25.9877, -31.0037) -> (25.6793, -31.2097) projected
  line L214 (25.6793, -31.2097) -> (25.3462, -31.3574) projected
  line L215 (25.3462, -31.3574) -> (25.0246, -31.5328) projected
  line L216 (25.0246, -31.5328) -> (24.8708, -31.6373) projected
  line L217 (24.8708, -31.6373) -> (24.7225, -31.7559) projected
  line L218 (24.7225, -31.7559) -> (24.5811, -31.892) projected
  line L219 (24.5811, -31.892) -> (24.4487, -32.0522) projected
  line L220 (24.4487, -32.0522) -> (24.3871, -32.145) projected
  line L221 (24.3871, -32.145) -> (24.3298, -32.2502) projected
  line L222 (24.3298, -32.2502) -> (24.279, -32.3741) projected
  line L223 (24.279, -32.3741) -> (24.2398, -32.5327) projected
  line L224 (24.2398, -32.5327) -> (24.2664, -32.892) projected
  line L225 (24.2664, -32.892) -> (24.4757, -33.6058) projected
  line L226 (24.4757, -33.6058) -> (24.6412, -34.3311) projected
  line L227 (24.6412, -34.3311) -> (24.7932, -34.6577) projected
  line L228 (24.7932, -34.6577) -> (24.9047, -34.777) projected
  line L229 (24.9047, -34.777) -> (25.0095, -34.8603) projected
  line L230 (25.0095, -34.8603) -> (25.1108, -34.9243) projected
  line L231 (25.1108, -34.9243) -> (25.2099, -34.9752) projected
  line L232 (25.2099, -34.9752) -> (25.4036, -35.0505) projected
  line L233 (25.4036, -35.0505) -> (25.5935, -35.1004) projected
  line L234 (25.5935, -35.1004) -> (25.7807, -35.1315) projected
  line L235 (25.7807, -35.1315) -> (25.966, -35.1478) projected
  line L236 (25.966, -35.1478) -> (26.3323, -35.144) projected
  line L237 (26.3323, -35.144) -> (26.6951, -35.1105) projected
  line L238 (26.6951, -35.1105) -> (27.0648, -35.1399) projected
  line L239 (27.0648, -35.1399) -> (27.4385, -35.2114) projected
  line L240 (27.4385, -35.2114) -> (27.8144, -35.3153) projected
  line L241 (27.8144, -35.3153) -> (28.1913, -35.4473) projected
  line L242 (28.1913, -35.4473) -> (28.5684, -35.6053) projected
  line L243 (28.5684, -35.6053) -> (28.9447, -35.7878) projected
  line L244 (28.9447, -35.7878) -> (29.3195, -35.9938) projected
  line L245 (29.3195, -35.9938) -> (29.692, -36.2224) projected
  line L246 (29.692, -36.2224) -> (30.0614, -36.4731) projected
  line L247 (30.0614, -36.4731) -> (30.3361, -36.6753) projected
  line L248 (30.3361, -36.6753) -> (30.2085, -38.8211) projected
  line L249 (30.2085, -38.8211) -> (29.9118, -38.9893) projected
  line L250 (29.9118, -38.9893) -> (29.5152, -39.1944) projected
  line L251 (29.5152, -39.1944) -> (29.1183, -39.3773) projected
  line L252 (29.1183, -39.3773) -> (28.7217, -39.5374) projected
  line L253 (28.7217, -39.5374) -> (28.3264, -39.674) projected
  line L254 (28.3264, -39.674) -> (27.9333, -39.7862) projected
  line L255 (27.9333, -39.7862) -> (27.5434, -39.8726) projected
  line L256 (27.5434, -39.8726) -> (27.1579, -39.9312) projected
  line L257 (27.1579, -39.9312) -> (26.7783, -39.958) projected
  line L258 (26.7783, -39.958) -> (26.4077, -39.9433) projected
  line L259 (26.4077, -39.9433) -> (26.0514, -39.867) projected
  line L260 (26.0514, -39.867) -> (25.6882, -39.8199) projected
  line L261 (25.6882, -39.8199) -> (25.5023, -39.814) projected
  line L262 (25.5023, -39.814) -> (25.3126, -39.8228) projected
  line L263 (25.3126, -39.8228) -> (25.1182, -39.8498) projected
  line L264 (25.1182, -39.8498) -> (24.9169, -39.9016) projected
  line L265 (24.9169, -39.9016) -> (24.8125, -39.9405) projected
  line L266 (24.8125, -39.9405) -> (24.7044, -39.9919) projected
  line L267 (24.7044, -39.9919) -> (24.5904, -40.0623) projected
  line L268 (24.5904, -40.0623) -> (24.4655, -40.1675) projected
  line L269 (24.4655, -40.1675) -> (24.2759, -40.4738) projected
  line L270 (24.2759, -40.4738) -> (24.0256, -41.1743) projected
  line L271 (24.0256, -41.1743) -> (23.7332, -41.8584) projected
  line L272 (23.7332, -41.8584) -> (23.6642, -42.2119) projected
  line L273 (23.6642, -42.2119) -> (23.6843, -42.3741) projected
  line L274 (23.6843, -42.3741) -> (23.7201, -42.5031) projected
  line L275 (23.7201, -42.5031) -> (23.7645, -42.6143) projected
  line L276 (23.7645, -42.6143) -> (23.8146, -42.7138) projected
  line L277 (23.8146, -42.7138) -> (23.9271, -42.8885) projected
  line L278 (23.9271, -42.8885) -> (24.0514, -43.0405) projected
  line L279 (24.0514, -43.0405) -> (24.1846, -43.1758) projected
  line L280 (24.1846, -43.1758) -> (24.325, -43.2978) projected
  line L281 (24.325, -43.2978) -> (24.6235, -43.5101) projected
  line L282 (24.6235, -43.5101) -> (24.9367, -43.6962) projected
  line L283 (24.9367, -43.6962) -> (25.2186, -43.9373) projected
  line L284 (25.2186, -43.9373) -> (25.4788, -44.2149) projected
  line L285 (25.4788, -44.2149) -> (25.7219, -44.5198) projected
  line L286 (25.7219, -44.5198) -> (25.9492, -44.8482) projected
  line L287 (25.9492, -44.8482) -> (26.1614, -45.1976) projected
  line L288 (26.1614, -45.1976) -> (26.3585, -45.5664) projected
  line L289 (26.3585, -45.5664) -> (26.5407, -45.9534) projected
  line L290 (26.5407, -45.9534) -> (26.7077, -46.3573) projected
  line L291 (26.7077, -46.3573) -> (26.8592, -46.7773) projected
  line L292 (26.8592, -46.7773) -> (26.9625, -47.1023) projected
  line L293 (26.9625, -47.1023) -> (25.5981, -48.7632) projected
  line L294 (25.5981, -48.7632) -> (25.2592, -48.7249) projected
  line L295 (25.2592, -48.7249) -> (24.8178, -48.6578) projected
  line L296 (24.8178, -48.6578) -> (24.3891, -48.5724) projected
  line L297 (24.3891, -48.5724) -> (23.9742, -48.4688) projected
  line L298 (23.9742, -48.4688) -> (23.5741, -48.347) projected
  line L299 (23.5741, -48.347) -> (23.1901, -48.2067) projected
  line L300 (23.1901, -48.2067) -> (22.8239, -48.0475) projected
  line L301 (22.8239, -48.0475) -> (22.4775, -47.8682) projected
  line L302 (22.4775, -47.8682) -> (22.1548, -47.6668) projected
  line L303 (22.1548, -47.6668) -> (21.8636, -47.4371) projected
  line L304 (21.8636, -47.4371) -> (21.6201, -47.166) projected
  line L305 (21.6201, -47.166) -> (21.354, -46.9143) projected
  line L306 (21.354, -46.9143) -> (21.207, -46.8003) projected
  line L307 (21.207, -46.8003) -> (21.0484, -46.696) projected
  line L308 (21.0484, -46.696) -> (20.8752, -46.6035) projected
  line L309 (20.8752, -46.6035) -> (20.682, -46.5271) projected
  line L310 (20.682, -46.5271) -> (20.5747, -46.4972) projected
  line L311 (20.5747, -46.4972) -> (20.4569, -46.4753) projected
  line L312 (20.4569, -46.4753) -> (20.3234, -46.4652) projected
  line L313 (20.3234, -46.4652) -> (20.1605, -46.4769) projected
  line L314 (20.1605, -46.4769) -> (19.827, -46.6133) projected
  line L315 (19.827, -46.6133) -> (19.2128, -47.0328) projected
  line L316 (19.2128, -47.0328) -> (18.5742, -47.4144) projected
  line L317 (18.5742, -47.4144) -> (18.3105, -47.6599) projected
  line L318 (18.3105, -47.6599) -> (18.2315, -47.8028) projected
  line L319 (18.2315, -47.8028) -> (18.1846, -47.9283) projected
  line L320 (18.1846, -47.9283) -> (18.1551, -48.0444) projected
  line L321 (18.1551, -48.0444) -> (18.1373, -48.1543) projected
  line L322 (18.1373, -48.1543) -> (18.1256, -48.3618) projected
  line L323 (18.1256, -48.3618) -> (18.1368, -48.5578) projected
  line L324 (18.1368, -48.5578) -> (18.165, -48.7455) projected
  line L325 (18.165, -48.7455) -> (18.2068, -48.9267) projected
  line L326 (18.2068, -48.9267) -> (18.3236, -49.2739) projected
  line L327 (18.3236, -49.2739) -> (18.4675, -49.6086) projected
  line L328 (18.4675, -49.6086) -> (18.5539, -49.9694) projected
  line L329 (18.5539, -49.9694) -> (18.6013, -50.3469) projected
  line L330 (18.6013, -50.3469) -> (18.6187, -50.7364) projected
  line L331 (18.6187, -50.7364) -> (18.6096, -51.1357) projected
  line L332 (18.6096, -51.1357) -> (18.5758, -51.5431) projected
  line L333 (18.5758, -51.5431) -> (18.5186, -51.9574) projected
  line L334 (18.5186, -51.9574) -> (18.4385, -52.3775) projected
  line L335 (18.4385, -52.3775) -> (18.3362, -52.8024) projected
  line L336 (18.3362, -52.8024) -> (18.2119, -53.2313) projected
  line L337 (18.2119, -53.2313) -> (18.1045, -53.555) projected
  line L338 (18.1045, -53.555) -> (16.0243, -54.0967) projected
  line L339 (16.0243, -54.0967) -> (15.7727, -53.8665) projected
  line L340 (15.7727, -53.8665) -> (15.455, -53.5527) projected
  line L341 (15.455, -53.5527) -> (15.1584, -53.2317) projected
  line L342 (15.1584, -53.2317) -> (14.8836, -52.904) projected
  line L343 (14.8836, -52.904) -> (14.6315, -52.5703) projected
  line L344 (14.6315, -52.5703) -> (14.4034, -52.2311) projected
  line L345 (14.4034, -52.2311) -> (14.2006, -51.887) projected
  line L346 (14.2006, -51.887) -> (14.0258, -51.5384) projected
  line L347 (14.0258, -51.5384) -> (13.8831, -51.1857) projected
  line L348 (13.8831, -51.1857) -> (13.7825, -50.8287) projected
  line L349 (13.7825, -50.8287) -> (13.7449, -50.4663) projected
  line L350 (13.7449, -50.4663) -> (13.6775, -50.1063) projected
  line L351 (13.6775, -50.1063) -> (13.6256, -49.9276) projected
  line L352 (13.6256, -49.9276) -> (13.5587, -49.75) projected
  line L353 (13.5587, -49.75) -> (13.4729, -49.5734) projected
  line L354 (13.4729, -49.5734) -> (13.3615, -49.398) projected
  line L355 (13.3615, -49.398) -> (13.2922, -49.3107) projected
  line L356 (13.2922, -49.3107) -> (13.2099, -49.2238) projected
  line L357 (13.2099, -49.2238) -> (13.1078, -49.1372) projected
  line L358 (13.1078, -49.1372) -> (12.9691, -49.0509) projected
  line L359 (12.9691, -49.0509) -> (12.6192, -48.9652) projected
  line L360 (12.6192, -48.9652) -> (11.8756, -48.9436) projected
  line L361 (11.8756, -48.9436) -> (11.1347, -48.8769) projected
  line L362 (11.1347, -48.8769) -> (10.7771, -48.9205) projected
  line L363 (10.7771, -48.9205) -> (10.6291, -48.9898) projected
  line L364 (10.6291, -48.9898) -> (10.5175, -49.0637) projected
  line L365 (10.5175, -49.0637) -> (10.4254, -49.1402) projected
  line L366 (10.4254, -49.1402) -> (10.3463, -49.2187) projected
  line L367 (10.3463, -49.2187) -> (10.2149, -49.3797) projected
  line L368 (10.2149, -49.3797) -> (10.1088, -49.5448) projected
  line L369 (10.1088, -49.5448) -> (10.0213, -49.7133) projected
  line L370 (10.0213, -49.7133) -> (9.9486, -49.8845) projected
  line L371 (9.9486, -49.8845) -> (9.8389, -50.234) projected
  line L372 (9.8389, -50.234) -> (9.7587, -50.5894) projected
  line L373 (9.7587, -50.5894) -> (9.6165, -50.932) projected
  line L374 (9.6165, -50.932) -> (9.433, -51.2653) projected
  line L375 (9.433, -51.2653) -> (9.3025, -51.4628) projected
  arc A8 (9.3025, -51.4628) -> (-11.8073, -35.0555) centre (-30.819, -81.3) ccw projected
  arc A9 (-11.8073, -35.0555) -> (-3.2188, -28.9967) centre (-30.9527, 1.1999) ccw projected
  arc A10 (27.6302, -28.9967) -> (-3.2188, -28.9967) centre (12.2057, -45.7908) ccw projected
  circle A11 centre (19.3845, -32.452) radius 1.6 projected
  circle A12 centre (12.6039, -36.6975) radius 2.5 projected
  circle A13 centre (16.8493, -43.478) radius 1.6 projected
  circle A14 centre (5.8233, -40.9429) radius 1.6 projected
  circle A15 centre (8.3584, -29.9169) radius 1.6 projected
  line L376 (5.1017, -49.7257) -> (-11.8073, -49.7257)
  line L377 (-11.8073, -35.0555) -> (-11.8073, -49.7257)
  line L378 (9.3025, -51.4628) -> (-11.8073, -51.4628)
  line L379 (-11.8073, -51.4628) -> (-11.8073, -49.7257)
  point P0 (0, 0)
  point P1 (-11.8073, -35.0555)
  constraints: 12 end point, 3 perpendicular, 2 horizontal
extrude "Выдавливание2" add sketch "Эскиз2" against normal up to surface (5 mm away) contours A8 L378 L379 L377